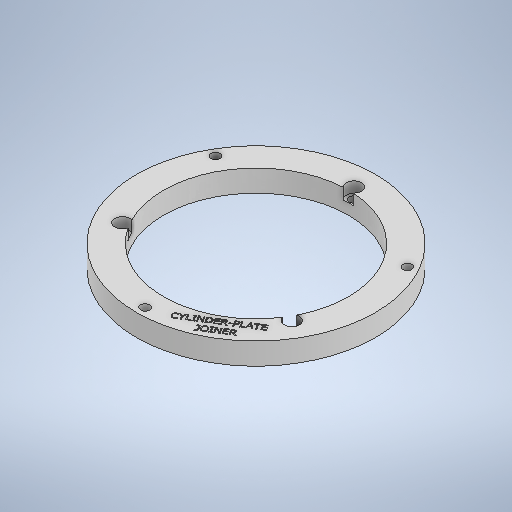
# Autodesk Inventor part: Cylinder-Plate Joiner
Saved by Autodesk Inventor 2025 (Build 290162000, 162)
## iProperties
Created: 2025-07-11
Part Number: Cylinder-Plate Joiner
Material: Generic
Document SubType Name: Modeling
Designer: mumin
Density: 1 g/cm^3
Appearance: Default
Author: mumin
Autodesk Inventor part; units mm, degrees
ref_plane "YZ Plane" through (0, 0, 0) normal (1, 0, 0) x (0, 1, 0)
ref_plane "XZ Plane" through (0, 0, 0) normal (0, 1, 0) x (-1, 0, 0)
ref_plane "XY Plane" through (0, 0, 0) normal (0, 0, 1) x (1, 0, 0)
sketch "Sketch1" plane through (0, 0, 0) normal (0, 1, 0) x (-1, 0, 0)
  circle A0 centre (0, 0) radius 42.5
  circle A1 centre (0, 0) radius 55
  dimension "d0" = 85
  dimension "d1" = 110
  constraints: 2 centre point, 2 coincident
  measures "d0" diameter of A0
  measures "d1" diameter of A1
extrude "Extrusion1" add sketch "Sketch1" along normal blind 10
sketch "Sketch2" plane through (0, 10, 0) normal (0, 1, 0) x (1, 0, 0)
  line L0 (0, 77) -> (0, -77) projected
  point P0 (0, 0)
  point P1 (0, 45)
  dimension "d13" = 45
  constraints: 1 point on line
  measures "d13" distance of point (0, 0) point (0, 45)
hole "Cylinder Mounts" at (0, 10, -45) direction (0, -1, 0) diameter 4.2 end through all counterbore diameter 7 counterbore depth 5
pattern_circular "Circular Pattern1" count 3 over 360 about axis through (0, -10, 0) along (0, 1, 0) of "Cylinder Mounts"
sketch "Sketch3" plane through (0, 0, 0) normal (0, -1, 0) x (1, 0, 0)
  line L0 (0, -77) -> (0, 77) projected
  point P0 (0, 0)
  point P1 (0, 51)
  dimension "d24" = 51
  constraints: 1 point on line
  measures "d24" distance of point (0, 0) point (0, 51)
hole "Head Plate Mounts" at (0, 0, 51) direction (0, 1, 0) diameter 4.2 end through all counterbore diameter 7 counterbore depth 5
pattern_circular "Circular Pattern2" count 3 over 360 about axis through (0, -10, 0) along (0, 1, 0) of "Head Plate Mounts"
sketch "Sketch4" plane through (0, 10, 0) normal (0, 1, 0) x (1, 0, 0)
  line L0 (1.5624, -50.7881) -> (42.0552, -25.4952) construction
  line L1 (42.0552, -25.4952) -> (43.738, -28.1893) construction
  line L2 (43.738, -28.1893) -> (3.2452, -53.4821) construction
  line L3 (3.2452, -53.4821) -> (1.5624, -50.7881) construction
  spline S0 degree 2 poles (11.0101, -48.6087) (10.7587, -48.7657) (10.2274, -48.8617) (9.9664, -48.7888) knots 0 0 0 1 2 2 2
  spline S1 degree 2 poles (9.9664, -48.7888) (9.7067, -48.7181) (9.223, -48.3213) (9.0188, -47.9945) knots 0 0 0 1 2 2 2
  spline S2 degree 2 poles (9.0188, -47.9945) (8.816, -47.6698) (8.6805, -47.0846) (8.7264, -46.8083) knots 0 0 0 1 2 2 2
  spline S3 degree 2 poles (8.7264, -46.8083) (8.7728, -46.5376) (9.0822, -46.091) (9.344, -45.9275) knots 0 0 0 1 2 2 2
  spline S4 degree 2 poles (9.344, -45.9275) (9.4739, -45.8464) (9.7258, -45.7414) (9.8405, -45.7106) knots 0 0 0 1 2 2 2
  spline S5 degree 2 poles (9.8405, -45.7106) (9.9413, -45.6855) (10.1636, -45.6544) (10.2783, -45.6468) knots 0 0 0 1 2 2 2
  line L4 (10.2783, -45.6468) -> (10.5374, -46.0616)
  line L5 (10.5374, -46.0616) -> (10.5101, -46.0786)
  spline S6 degree 2 poles (10.5101, -46.0786) (10.4379, -46.0655) (10.2222, -46.0372) (10.0842, -46.0447) knots 0 0 0 1 2 2 2
  spline S7 degree 2 poles (10.0842, -46.0447) (9.9517, -46.0517) (9.676, -46.1279) (9.5251, -46.2221) knots 0 0 0 1 2 2 2
  spline S8 degree 2 poles (9.5251, -46.2221) (9.3596, -46.3255) (9.1493, -46.6461) (9.1194, -46.8454) knots 0 0 0 1 2 2 2
  spline S9 degree 2 poles (9.1194, -46.8454) (9.0929, -47.0454) (9.2213, -47.5214) (9.3771, -47.7707) knots 0 0 0 1 2 2 2
  spline S10 degree 2 poles (9.3771, -47.7707) (9.5432, -48.0368) (9.9105, -48.3403) (10.104, -48.4029) knots 0 0 0 1 2 2 2
  spline S11 degree 2 poles (10.104, -48.4029) (10.2927, -48.4627) (10.665, -48.4107) (10.8284, -48.3086) knots 0 0 0 1 2 2 2
  spline S12 degree 2 poles (10.8284, -48.3086) (10.9772, -48.2157) (11.1849, -47.9841) (11.2493, -47.8681) knots 0 0 0 1 2 2 2
  spline S13 degree 2 poles (11.2493, -47.8681) (11.3096, -47.7547) (11.3793, -47.5539) (11.3942, -47.4893) knots 0 0 0 1 2 2 2
  line L6 (11.3942, -47.4893) -> (11.4193, -47.4736)
  line L7 (11.4193, -47.4736) -> (11.6758, -47.8842)
  spline S14 degree 2 poles (11.6758, -47.8842) (11.6148, -47.9776) (11.5097, -48.1452) (11.4238, -48.2454) knots 0 0 0 1 2 2 2
  spline S15 degree 2 poles (11.4238, -48.2454) (11.3343, -48.3538) (11.1651, -48.5119) (11.0101, -48.6087) knots 0 0 0 1 2 2 2
  line L8 (12.3015, -44.1442) -> (12.3282, -46.1312)
  line L9 (12.3282, -46.1312) -> (13.0427, -47.275)
  line L10 (13.0427, -47.275) -> (12.6991, -47.4896)
  line L11 (12.6991, -47.4896) -> (12.0069, -46.3814)
  line L12 (12.0069, -46.3814) -> (10.2108, -45.4502)
  line L13 (10.2108, -45.4502) -> (10.5921, -45.212)
  line L14 (10.5921, -45.212) -> (11.9709, -45.9321)
  line L15 (11.9709, -45.9321) -> (11.937, -44.3719)
  line L16 (11.937, -44.3719) -> (12.3015, -44.1442)
  line L17 (15.653, -45.6446) -> (14.1551, -46.5802)
  line L18 (14.1551, -46.5802) -> (12.5403, -43.9951)
  line L19 (12.5403, -43.9951) -> (12.8839, -43.7805)
  line L20 (12.8839, -43.7805) -> (14.3076, -46.0597)
  line L21 (14.3076, -46.0597) -> (15.4619, -45.3387)
  line L22 (15.4619, -45.3387) -> (15.653, -45.6446)
  line L23 (16.824, -44.9131) -> (15.8226, -45.5386)
  line L24 (15.8226, -45.5386) -> (15.6578, -45.2746)
  line L25 (15.6578, -45.2746) -> (15.9867, -45.0692)
  line L26 (15.9867, -45.0692) -> (14.7017, -43.012)
  line L27 (14.7017, -43.012) -> (14.3728, -43.2174)
  line L28 (14.3728, -43.2174) -> (14.2079, -42.9535)
  line L29 (14.2079, -42.9535) -> (15.2093, -42.328)
  line L30 (15.2093, -42.328) -> (15.3741, -42.5919)
  line L31 (15.3741, -42.5919) -> (15.0452, -42.7974)
  line L32 (15.0452, -42.7974) -> (16.3302, -44.8546)
  line L33 (16.3302, -44.8546) -> (16.6591, -44.6491)
  line L34 (16.6591, -44.6491) -> (16.824, -44.9131)
  line L35 (19.0991, -43.492) -> (18.7136, -43.7328)
  line L36 (18.7136, -43.7328) -> (16.1775, -42.2183)
  line L37 (16.1775, -42.2183) -> (17.5698, -44.4473)
  line L38 (17.5698, -44.4473) -> (17.2493, -44.6475)
  line L39 (17.2493, -44.6475) -> (15.6345, -42.0623)
  line L40 (15.6345, -42.0623) -> (16.1227, -41.7574)
  line L41 (16.1227, -41.7574) -> (18.4423, -43.1538)
  line L42 (18.4423, -43.1538) -> (17.1638, -41.1071)
  line L43 (17.1638, -41.1071) -> (17.4844, -40.9069)
  line L44 (17.4844, -40.9069) -> (19.0991, -43.492)
  spline S16 degree 2 poles (20.8551, -40.6012) (21.0763, -40.9552) (21.1452, -41.7043) (21.0037, -42.014) knots 0 0 0 1 2 2 2
  spline S17 degree 2 poles (21.0037, -42.014) (20.884, -42.2606) (20.532, -42.597) (20.2178, -42.7933) knots 0 0 0 1 2 2 2
  line L45 (20.2178, -42.7933) -> (19.6228, -43.1649)
  line L46 (19.6228, -43.1649) -> (18.0081, -40.5798)
  line L47 (18.0081, -40.5798) -> (18.5968, -40.2121)
  spline S18 degree 2 poles (18.5968, -40.2121) (18.9613, -39.9844) (19.4441, -39.8342) (19.651, -39.839) knots 0 0 0 1 2 2 2
  spline S19 degree 2 poles (19.651, -39.839) (20.0036, -39.8488) (20.6196, -40.2241) (20.8551, -40.6012) knots 0 0 0 1 2 2 2
  spline S20 degree 2 poles (20.4943, -40.8208) (20.3085, -40.5233) (19.8485, -40.2252) (19.5791, -40.2275) knots 0 0 0 1 2 2 2
  spline S21 degree 2 poles (19.5791, -40.2275) (19.3898, -40.2322) (19.0319, -40.3538) (18.7993, -40.4991) knots 0 0 0 1 2 2 2
  line L48 (18.7993, -40.4991) -> (18.5375, -40.6626)
  line L49 (18.5375, -40.6626) -> (19.7806, -42.6528)
  line L50 (19.7806, -42.6528) -> (20.0424, -42.4892)
  spline S22 degree 2 poles (20.0424, -42.4892) (20.2708, -42.3466) (20.5707, -42.0574) (20.6495, -41.8712) knots 0 0 0 1 2 2 2
  spline S23 degree 2 poles (20.6495, -41.8712) (20.7538, -41.6372) (20.6827, -41.1224) (20.4943, -40.8208) knots 0 0 0 1 2 2 2
  line L51 (22.0341, -41.6588) -> (20.4193, -39.0736)
  line L52 (20.4193, -39.0736) -> (22.0366, -38.0634)
  line L53 (22.0366, -38.0634) -> (22.2277, -38.3693)
  line L54 (22.2277, -38.3693) -> (20.954, -39.1649)
  line L55 (20.954, -39.1649) -> (21.3962, -39.873)
  line L56 (21.3962, -39.873) -> (22.5841, -39.131)
  line L57 (22.5841, -39.131) -> (22.7751, -39.4369)
  line L58 (22.7751, -39.4369) -> (21.5873, -40.1788)
  line L59 (21.5873, -40.1788) -> (22.1866, -41.1383)
  line L60 (22.1866, -41.1383) -> (23.4603, -40.3427)
  line L61 (23.4603, -40.3427) -> (23.6514, -40.6486)
  line L62 (23.6514, -40.6486) -> (22.0341, -41.6588)
  line L63 (26.0291, -39.1634) -> (25.5829, -39.4421)
  line L64 (25.5829, -39.4421) -> (24.1234, -38.9238)
  line L65 (24.1234, -38.9238) -> (23.7295, -39.1698)
  line L66 (23.7295, -39.1698) -> (24.372, -40.1984)
  line L67 (24.372, -40.1984) -> (24.0284, -40.413)
  line L68 (24.0284, -40.413) -> (22.4137, -37.8279)
  line L69 (22.4137, -37.8279) -> (23.0799, -37.4118)
  spline S24 degree 2 poles (23.0799, -37.4118) (23.302, -37.2731) (23.6316, -37.1341) (23.8227, -37.1371) knots 0 0 0 1 2 2 2
  spline S25 degree 2 poles (23.8227, -37.1371) (24.0139, -37.14) (24.3424, -37.3163) (24.4693, -37.5195) knots 0 0 0 1 2 2 2
  spline S26 degree 2 poles (24.4693, -37.5195) (24.646, -37.8023) (24.5964, -38.3663) (24.4067, -38.6128) knots 0 0 0 1 2 2 2
  line L70 (24.4067, -38.6128) -> (26.0291, -39.1634)
  spline S27 degree 2 poles (24.1281, -37.7705) (24.0575, -37.6574) (23.8692, -37.5332) (23.7501, -37.529) knots 0 0 0 1 2 2 2
  spline S28 degree 2 poles (23.7501, -37.529) (23.6467, -37.5266) (23.427, -37.6085) (23.2846, -37.6975) knots 0 0 0 1 2 2 2
  line L71 (23.2846, -37.6975) -> (22.9431, -37.9108)
  line L72 (22.9431, -37.9108) -> (23.5502, -38.8828)
  line L73 (23.5502, -38.8828) -> (23.8519, -38.6944)
  spline S29 degree 2 poles (23.8519, -38.6944) (24.0007, -38.6015) (24.2047, -38.4012) (24.2353, -38.2685) knots 0 0 0 1 2 2 2
  spline S30 degree 2 poles (24.2353, -38.2685) (24.2663, -38.1502) (24.2119, -37.9046) (24.1281, -37.7705) knots 0 0 0 1 2 2 2
  line L74 (26.4995, -37.5153) -> (25.5212, -38.1264)
  line L75 (25.5212, -38.1264) -> (25.3249, -37.8122)
  line L76 (25.3249, -37.8122) -> (26.3032, -37.2011)
  line L77 (26.3032, -37.2011) -> (26.4995, -37.5153)
  spline S31 degree 2 poles (28.0309, -35.4026) (28.1356, -35.5702) (28.2046, -35.9464) (28.1632, -36.1179) knots 0 0 0 1 2 2 2
  spline S32 degree 2 poles (28.1632, -36.1179) (28.1116, -36.3336) (27.8342, -36.6962) (27.5577, -36.8689) knots 0 0 0 1 2 2 2
  line L78 (27.5577, -36.8689) -> (27.2665, -37.0508)
  line L79 (27.2665, -37.0508) -> (27.8684, -38.0145)
  line L80 (27.8684, -38.0145) -> (27.5249, -38.2291)
  line L81 (27.5249, -38.2291) -> (25.9101, -35.6439)
  line L82 (25.9101, -35.6439) -> (26.5596, -35.2383)
  spline S33 degree 2 poles (26.5596, -35.2383) (26.79, -35.0943) (27.1597, -34.9682) (27.337, -34.9769) knots 0 0 0 1 2 2 2
  spline S34 degree 2 poles (27.337, -34.9769) (27.543, -34.9851) (27.8962, -35.1868) (28.0309, -35.4026) knots 0 0 0 1 2 2 2
  spline S35 degree 2 poles (27.6793, -35.6368) (27.5955, -35.5027) (27.3803, -35.3634) (27.2468, -35.3594) knots 0 0 0 1 2 2 2
  spline S36 degree 2 poles (27.2468, -35.3594) (27.1311, -35.356) (26.8857, -35.4481) (26.7244, -35.5488) knots 0 0 0 1 2 2 2
  line L83 (26.7244, -35.5488) -> (26.4395, -35.7268)
  line L84 (26.4395, -35.7268) -> (27.0833, -36.7575)
  line L85 (27.0833, -36.7575) -> (27.3179, -36.6109)
  spline S37 degree 2 poles (27.3179, -36.6109) (27.5274, -36.4801) (27.7432, -36.2521) (27.7721, -36.1118) knots 0 0 0 1 2 2 2
  spline S38 degree 2 poles (27.7721, -36.1118) (27.8012, -35.9858) (27.7565, -35.7604) (27.6793, -35.6368) knots 0 0 0 1 2 2 2
  line L86 (30.9836, -36.0687) -> (29.4857, -37.0043)
  line L87 (29.4857, -37.0043) -> (27.871, -34.4191)
  line L88 (27.871, -34.4191) -> (28.2145, -34.2045)
  line L89 (28.2145, -34.2045) -> (29.6382, -36.4838)
  line L90 (29.6382, -36.4838) -> (30.7925, -35.7628)
  line L91 (30.7925, -35.7628) -> (30.9836, -36.0687)
  line L92 (30.9752, -36.0739) -> (30.2319, -32.9444)
  line L93 (30.2319, -32.9444) -> (30.6551, -32.6801)
  line L94 (30.6551, -32.6801) -> (33.1414, -34.7209)
  line L95 (33.1414, -34.7209) -> (32.7789, -34.9472)
  line L96 (32.7789, -34.9472) -> (32.0929, -34.371)
  line L97 (32.0929, -34.371) -> (31.1061, -34.9874)
  line L98 (31.1061, -34.9874) -> (31.323, -35.8567)
  line L99 (31.323, -35.8567) -> (30.9752, -36.0739)
  line L100 (31.8154, -34.1366) -> (30.655, -33.1694)
  line L101 (30.655, -33.1694) -> (31.0172, -34.6352)
  line L102 (31.0172, -34.6352) -> (31.8154, -34.1366)
  line L103 (33.9898, -34.1909) -> (32.5661, -31.9116)
  line L104 (32.5661, -31.9116) -> (31.6988, -32.4534)
  line L105 (31.6988, -32.4534) -> (31.5078, -32.1475)
  line L106 (31.5078, -32.1475) -> (33.5859, -30.8494)
  line L107 (33.5859, -30.8494) -> (33.777, -31.1553)
  line L108 (33.777, -31.1553) -> (32.9097, -31.697)
  line L109 (32.9097, -31.697) -> (34.3334, -33.9763)
  line L110 (34.3334, -33.9763) -> (33.9898, -34.1909)
  line L111 (35.4625, -33.271) -> (33.8478, -30.6859)
  line L112 (33.8478, -30.6859) -> (35.4651, -29.6757)
  line L113 (35.4651, -29.6757) -> (35.6561, -29.9815)
  line L114 (35.6561, -29.9815) -> (34.3824, -30.7771)
  line L115 (34.3824, -30.7771) -> (34.8247, -31.4852)
  line L116 (34.8247, -31.4852) -> (36.0125, -30.7433)
  line L117 (36.0125, -30.7433) -> (36.2036, -31.0491)
  line L118 (36.2036, -31.0491) -> (35.0157, -31.7911)
  line L119 (35.0157, -31.7911) -> (35.615, -32.7505)
  line L120 (35.615, -32.7505) -> (36.8888, -31.9549)
  line L121 (36.8888, -31.9549) -> (37.0798, -32.2608)
  line L122 (37.0798, -32.2608) -> (35.4625, -33.271)
  spline S39 degree 2 poles (20.9784, -47.3003) (21.1904, -47.6397) (21.0059, -48.2675) (20.656, -48.486) knots 0 0 0 1 2 2 2
  spline S40 degree 2 poles (20.656, -48.486) (20.5723, -48.5384) (20.2753, -48.6831) (20.168, -48.721) knots 0 0 0 1 2 2 2
  line L123 (20.168, -48.721) -> (19.9612, -48.39)
  line L124 (19.9612, -48.39) -> (19.9801, -48.3782)
  spline S41 degree 2 poles (19.9801, -48.3782) (20.067, -48.3589) (20.3152, -48.2854) (20.4241, -48.2173) knots 0 0 0 1 2 2 2
  spline S42 degree 2 poles (20.4241, -48.2173) (20.5834, -48.1179) (20.7282, -47.9255) (20.7303, -47.831) knots 0 0 0 1 2 2 2
  spline S43 degree 2 poles (20.7303, -47.831) (20.7353, -47.7317) (20.6348, -47.5149) (20.5524, -47.3829) knots 0 0 0 1 2 2 2
  line L125 (20.5524, -47.3829) -> (19.6116, -45.8767)
  line L126 (19.6116, -45.8767) -> (19.0648, -46.2182)
  line L127 (19.0648, -46.2182) -> (18.8934, -45.9438)
  line L128 (18.8934, -45.9438) -> (19.7837, -45.3877)
  line L129 (19.7837, -45.3877) -> (20.9784, -47.3003)
  spline S44 degree 2 poles (22.304, -44.224) (22.558, -44.3042) (23.0354, -44.7049) (23.237, -45.0275) knots 0 0 0 1 2 2 2
  spline S45 degree 2 poles (23.237, -45.0275) (23.4332, -45.3418) (23.592, -45.9503) (23.5485, -46.2163) knots 0 0 0 1 2 2 2
  spline S46 degree 2 poles (23.5485, -46.2163) (23.5018, -46.4959) (23.188, -46.9307) (22.9345, -47.089) knots 0 0 0 1 2 2 2
  spline S47 degree 2 poles (22.9345, -47.089) (22.6727, -47.2526) (22.1425, -47.3362) (21.8809, -47.2579) knots 0 0 0 1 2 2 2
  spline S48 degree 2 poles (21.8809, -47.2579) (21.6249, -47.179) (21.1503, -46.7736) (20.9514, -46.4552) knots 0 0 0 1 2 2 2
  spline S49 degree 2 poles (20.9514, -46.4552) (20.7486, -46.1304) (20.6011, -45.5353) (20.6386, -45.2643) knots 0 0 0 1 2 2 2
  spline S50 degree 2 poles (20.6386, -45.2643) (20.6821, -44.9983) (20.992, -44.5572) (21.2517, -44.395) knots 0 0 0 1 2 2 2
  spline S51 degree 2 poles (21.2517, -44.395) (21.5157, -44.2301) (22.054, -44.1501) (22.304, -44.224) knots 0 0 0 1 2 2 2
  spline S52 degree 2 poles (22.8787, -45.2513) (22.7191, -44.9957) (22.3607, -44.6691) (22.1791, -44.6021) knots 0 0 0 1 2 2 2
  spline S53 degree 2 poles (22.1791, -44.6021) (21.9927, -44.5321) (21.6198, -44.5786) (21.4397, -44.6911) knots 0 0 0 1 2 2 2
  spline S54 degree 2 poles (21.4397, -44.6911) (21.2532, -44.8076) (21.0536, -45.1128) (21.0331, -45.3178) knots 0 0 0 1 2 2 2
  spline S55 degree 2 poles (21.0331, -45.3178) (21.0129, -45.5139) (21.1526, -45.98) (21.3096, -46.2314) knots 0 0 0 1 2 2 2
  spline S56 degree 2 poles (21.3096, -46.2314) (21.6276, -46.7405) (22.3926, -47.014) (22.7508, -46.7902) knots 0 0 0 1 2 2 2
  spline S57 degree 2 poles (22.7508, -46.7902) (23.109, -46.5665) (23.1967, -45.7604) (22.8787, -45.2513) knots 0 0 0 1 2 2 2
  line L130 (25.3222, -45.5219) -> (24.3209, -46.1474)
  line L131 (24.3209, -46.1474) -> (24.156, -45.8834)
  line L132 (24.156, -45.8834) -> (24.4849, -45.678)
  line L133 (24.4849, -45.678) -> (23.1999, -43.6208)
  line L134 (23.1999, -43.6208) -> (22.871, -43.8262)
  line L135 (22.871, -43.8262) -> (22.7061, -43.5622)
  line L136 (22.7061, -43.5622) -> (23.7075, -42.9368)
  line L137 (23.7075, -42.9368) -> (23.8724, -43.2007)
  line L138 (23.8724, -43.2007) -> (23.5435, -43.4062)
  line L139 (23.5435, -43.4062) -> (24.8285, -45.4634)
  line L140 (24.8285, -45.4634) -> (25.1574, -45.2579)
  line L141 (25.1574, -45.2579) -> (25.3222, -45.5219)
  line L142 (27.5973, -44.1008) -> (27.2119, -44.3416)
  line L143 (27.2119, -44.3416) -> (24.6757, -42.827)
  line L144 (24.6757, -42.827) -> (26.068, -45.056)
  line L145 (26.068, -45.056) -> (25.7475, -45.2563)
  line L146 (25.7475, -45.2563) -> (24.1328, -42.6711)
  line L147 (24.1328, -42.6711) -> (24.6209, -42.3662)
  line L148 (24.6209, -42.3662) -> (26.9405, -43.7626)
  line L149 (26.9405, -43.7626) -> (25.6621, -41.7159)
  line L150 (25.6621, -41.7159) -> (25.9826, -41.5157)
  line L151 (25.9826, -41.5157) -> (27.5973, -44.1008)
  line L152 (28.1211, -43.7737) -> (26.5063, -41.1885)
  line L153 (26.5063, -41.1885) -> (28.1236, -40.1783)
  line L154 (28.1236, -40.1783) -> (28.3146, -40.4842)
  line L155 (28.3146, -40.4842) -> (27.0409, -41.2798)
  line L156 (27.0409, -41.2798) -> (27.4832, -41.9879)
  line L157 (27.4832, -41.9879) -> (28.671, -41.2459)
  line L158 (28.671, -41.2459) -> (28.8621, -41.5518)
  line L159 (28.8621, -41.5518) -> (27.6743, -42.2937)
  line L160 (27.6743, -42.2937) -> (28.2736, -43.2532)
  line L161 (28.2736, -43.2532) -> (29.5473, -42.4576)
  line L162 (29.5473, -42.4576) -> (29.7383, -42.7635)
  line L163 (29.7383, -42.7635) -> (28.1211, -43.7737)
  line L164 (32.1161, -41.2783) -> (31.6698, -41.557)
  line L165 (31.6698, -41.557) -> (30.2103, -41.0387)
  line L166 (30.2103, -41.0387) -> (29.8165, -41.2847)
  line L167 (29.8165, -41.2847) -> (30.459, -42.3133)
  line L168 (30.459, -42.3133) -> (30.1154, -42.5279)
  line L169 (30.1154, -42.5279) -> (28.5007, -39.9428)
  line L170 (28.5007, -39.9428) -> (29.1669, -39.5267)
  spline S58 degree 2 poles (29.1669, -39.5267) (29.3889, -39.388) (29.7186, -39.249) (29.9097, -39.252) knots 0 0 0 1 2 2 2
  spline S59 degree 2 poles (29.9097, -39.252) (30.1008, -39.2549) (30.4294, -39.4312) (30.5563, -39.6344) knots 0 0 0 1 2 2 2
  spline S60 degree 2 poles (30.5563, -39.6344) (30.733, -39.9172) (30.6833, -40.4812) (30.4937, -40.7278) knots 0 0 0 1 2 2 2
  line L171 (30.4937, -40.7278) -> (32.1161, -41.2783)
  spline S61 degree 2 poles (30.2151, -39.8854) (30.1444, -39.7723) (29.9562, -39.6481) (29.8371, -39.6439) knots 0 0 0 1 2 2 2
  spline S62 degree 2 poles (29.8371, -39.6439) (29.7337, -39.6415) (29.514, -39.7234) (29.3715, -39.8124) knots 0 0 0 1 2 2 2
  line L172 (29.3715, -39.8124) -> (29.0301, -40.0257)
  line L173 (29.0301, -40.0257) -> (29.6372, -40.9977)
  line L174 (29.6372, -40.9977) -> (29.9389, -40.8093)
  spline S63 degree 2 poles (29.9389, -40.8093) (30.0876, -40.7164) (30.2916, -40.5162) (30.3223, -40.3834) knots 0 0 0 1 2 2 2
  spline S64 degree 2 poles (30.3223, -40.3834) (30.3532, -40.2651) (30.2988, -40.0195) (30.2151, -39.8854) knots 0 0 0 1 2 2 2
  point P0 (0, 0)
  constraints: 2 other
emboss "Emboss1" sketch "Sketch4" operation cut depth 1 direction (0, -1, 0)
body "Solid1"
